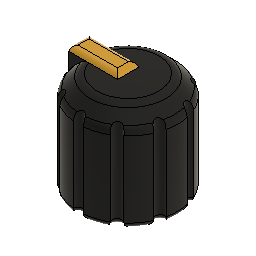
knob (Autodesk Fusion 360 design; units mm, degrees)
Autodesk Fusion 360 part; units mm, degrees
sketch "Sketch1" plane through (0, 0, 0) normal (0, 0, 1) x (1, 0, 0)
  circle A0 centre (0, 0) radius 3.1
  circle A1 centre (0, 0) radius 5
  circle A2 centre (0, 0) radius 3
  circle A3 centre (0, 5) radius 0.5
  circle A4 centre (-2.9389, 4.0451) radius 0.5
  circle A5 centre (-4.7553, 1.5451) radius 0.5
  circle A6 centre (-4.7553, -1.5451) radius 0.5
  circle A7 centre (-2.9389, -4.0451) radius 0.5
  circle A8 centre (0, -5) radius 0.5
  circle A9 centre (2.9389, -4.0451) radius 0.5
  circle A10 centre (4.7553, -1.5451) radius 0.5
  circle A11 centre (4.7553, 1.5451) radius 0.5
  circle A12 centre (2.9389, 4.0451) radius 0.5
  line L0 (0, 0) -> (0, 1.0451)
  line L1 (0, 1.0451) -> (-4.8896, 1.0451)
  line L2 (0, 0) -> (0, -1.0451)
  line L3 (0, -1.0451) -> (-4.8896, -1.0451)
  dimension "d1" = 6.2
  dimension "d2" = 10
  dimension "d3" = 6
  dimension "d4" = 1
  dimension "d6" = 360
  constraint coincident A0.centre A1.centre
  constraint concentric A0 A1
  constraint concentric A0 A2
  constraint coincident A1 A3.centre
  constraint vertical L0
  constraint horizontal L1
  constraint vertical L2
  constraint horizontal L3
  constraint coincident A1 L1.end
  constraint coincident A1 L3.end
  constraint tangent A6 L3
  constraint tangent A5 L1
  measures "d1" diameter of A0
  measures "d2" diameter of A1
  measures "d3" diameter of A2
  measures "d4" diameter of A3
extrude "Extrude1" add sketch "Sketch1" along normal blind 9 contours A0 A1 A3 A4 A5 A6 A7 A8 A9 A10 A11 A12 L1 L3 | A0 A1 L1 L3 | A1 A5 L1 | A1 A6 L3
extrude "Extrude2" add sketch "Sketch1" along normal blind 9 and the other way blind -4 contours A0 A2 L1 L3 | A0 A2 L1 L3
extrude "Extrude3" add sketch "Sketch1" along normal blind 1 from surface at 9 contours A0 A2 L1 L3 | A0 A1 A3 A4 A5 A6 A7 A8 A9 A10 A11 A12 L1 L3 | A0 A2 L1 L3 | A0 A1 L1 L3 | A2 L0 L1 L2 L3 | A2 L0 L1 L2 L3 | A1 A5 L1 | A1 A6 L3
sketch "Sketch2" plane through (0, 0, 0) normal (1, 0, 0) x (0, 1, 0)
  line L0 (-5.5, 8) -> (-3, 10.5)
  line L1 (-3, 10.5) -> (-5.5, 10.5)
  line L2 (-5.5, 10.5) -> (-5.5, 8)
  dimension "d26" = 8
  dimension "d27" = 3
  constraint horizontal L1
  constraint perpendicular L1 L2
  measures "d26" vertical distance of origin L0.start
  measures "d27" horizontal distance of origin L0.end
revolve "Revolve1" cut sketch "Sketch2" angle 360 about axis through (0, 0, 1.75) along (0, 0, 1)
fillet "Fillet4" radius 1 1 edges at (-1.2657, 3.2631, 10)
fillet "Fillet5" radius 1 10 edges at (4.0451, 2.9389, 8.5) (1.5451, 4.7553, 8.5) (-1.5451, 4.7553, 8.5) (-4.0451, 2.9389, 8.5) (-5, 0, 8.5) (-4.0451, -2.9389, 8.5) (-1.5451, -4.7553, 8.5) (1.5451, -4.7553, 8.5) (4.0451, -2.9389, 8.5) (5, 0, 8.5)
extrude "Extrude4" add sketch "Sketch1" along normal blind 10.5 and the other way blind -7.5 contours A0 A2 L1 L3 | A0 A1 L1 L3 | A2 L0 L1 L2 L3 picked at (-2.8875, 0.9086) picked at (-0.9374, 0.6967)
fillet "Fillet6" radius 0.5 4 edges at (-5, 0, 10.5) (-2.4448, -1.0451, 10.5) (0, 0, 10.5) (-2.4448, 1.0451, 10.5)
fillet "Fillet7" radius 0.5 1 faces at (4.2069, -0.4845, 0)
